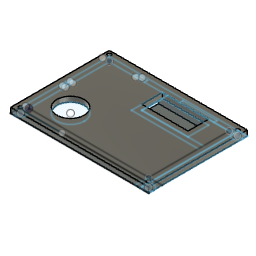
macronoxylid V2 v1 (Autodesk Fusion 360 design; units mm, degrees)
Autodesk Fusion 360 part; units mm, degrees
sketch "Sketch1" plane through (0, 0, 0) normal (0, 0, 1) x (1, 0, 0)
  line L0 (1, 0) -> (69, 0)
  line L1 (0, 1) -> (0, 46)
  line L2 (1, 47) -> (17.5, 47)
  line L3 (17.5, 47) -> (15.35, 47)
  line L4 (70, 1) -> (70, 46)
  line L5 (0, 23.5) -> (0, 25.65)
  line L6 (0, 23.5) -> (0, 21.35)
  line L7 (-1.7, 23.5) -> (-1.7, 25.8)
  line L8 (-1.7, 23.5) -> (-1.7, 21.2)
  line L9 (0, 0) -> (-2.8284, -2.8284)
  line L10 (0, 0) -> (-2, 0) construction
  line L11 (70, 47) -> (72.8284, 49.8284)
  line L12 (70, 47) -> (74, 47) construction
  line L13 (70, 0) -> (72.8284, -2.8284)
  line L14 (0, 47) -> (-2.8284, 49.8284)
  line L15 (0, 47) -> (-4, 47) construction
  line L16 (-2.8284, 49.8284) -> (72.8284, 49.8284)
  line L17 (72.8284, 49.8284) -> (72.8284, -2.8284)
  line L18 (72.8284, -2.8284) -> (-2.8284, -2.8284)
  line L19 (-2.8284, 49.8284) -> (-2.8284, -2.8284)
  line L20 (17.5, 47) -> (69, 47)
  line L21 (41.1957, 48.7475) -> (61.1957, 48.7475)
  line L22 (41.1957, 48.7475) -> (41.1957, 47)
  line L23 (61.1957, 48.7475) -> (61.1957, 47)
  line L24 (17.5, 48.7) -> (14.5, 48.7)
  line L25 (14.5, 48.7) -> (20.5, 48.7)
  line L26 (20.5, 48.7) -> (20.5, 47)
  line L27 (14.5, 48.7) -> (14.5, 47)
  line L28 (-1.7, 23.5) -> (-1.7, 26.5)
  line L29 (-1.7, 26.5) -> (-1.7, 23.5)
  line L30 (-1.7, 23.5) -> (-1.7, 20.5)
  line L31 (-1.7, 20.5) -> (-1.7, 26.5)
  line L32 (0, 26.5) -> (-1.7, 26.5)
  line L33 (-1.7, 20.5) -> (0, 20.5)
  arc A0 (70, 46) -> (69, 47) centre (70, 47) ccw
  arc A1 (1, 47) -> (0, 46) centre (0, 47) ccw
  arc A2 (0, 1) -> (1, 0) centre (0, 0) ccw
  arc A3 (69, 0) -> (70, 1) centre (70, 0) ccw
  line L34 (-2.8284, -2.8284) -> (22.1716, -2.8284)
  circle A4 centre (14.6716, 9.6716) radius 8
  line L35 (70, 47) -> (34, 47)
  line L36 (34, 47) -> (34, 32)
  line L37 (34, 32) -> (70, 32)
  line L38 (34, 32) -> (61, 32)
  line L39 (61, 32) -> (61, 44)
  line L40 (61, 44) -> (34, 44)
  line L41 (34, 44) -> (34, 32)
  line L42 (34, 47) -> (31, 47)
  line L43 (31, 47) -> (31, 29)
  line L44 (31, 29) -> (70, 29)
  line L45 (-2.8284, -2.8284) -> (72.8284, -2.8284)
  line L46 (72.8284, -2.8284) -> (72.8284, -7.8284)
  line L47 (72.8284, -7.8284) -> (-2.8284, -7.8284)
  line L48 (-2.8284, -7.8284) -> (-2.8284, -2.8284)
  line L49 (72.8284, -7.8284) -> (77.8284, -7.8284)
  line L50 (77.8284, -7.8284) -> (77.8284, 49.8284)
  line L51 (77.8284, 49.8284) -> (72.8284, 49.8284)
  line L52 (72.8284, 49.8284) -> (72.8284, -7.8284)
  line L53 (-2.8284, 49.8284) -> (-1.4496, 48.4496)
  circle A5 centre (-0.7071, 47.7071) radius 1.05
  line L54 (69, 47) -> (77.8284, 47)
  line L55 (69, 0) -> (77.8284, 0)
  line L56 (70, 0) -> (70, -7.8284)
  line L57 (0, 1) -> (0, -7.8284)
  line L58 (77.8284, -7.8284) -> (74.9994, -7.8284)
  line L59 (74.9994, -7.8284) -> (74.9994, 49.8284)
  line L60 (77.8284, -7.8284) -> (77.8284, -4.9994)
  line L61 (77.8284, -4.9994) -> (-2.8284, -4.9994)
  circle A6 centre (74.9994, 47) radius 2.829
  circle A7 centre (74.9994, -4.9994) radius 2.829
  circle A8 centre (0, -4.9994) radius 2.829
  circle A9 centre (0, -4.9994) radius 1.05
  circle A10 centre (74.9994, -4.9994) radius 1.05
  circle A11 centre (74.9994, 47) radius 1.05
  dimension "d1" = 70
  dimension "d2" = 47
  dimension "d3" = 17.5
  dimension "d5" = 2.15
  dimension "d23" = 2.15
  dimension "d25" = 1.7
  dimension "d26" = 2.3
  dimension "d27" = 2.3
  dimension "d28" = 45
  dimension "d29" = 4
  dimension "d30" = 4
  dimension "d31" = 45
  dimension "d32" = 4
  dimension "d33" = 45
  dimension "d34" = 4
  dimension "d59" = 6
  dimension "d60" = 3
  dimension "d61" = 3
  dimension "d62" = 2
  dimension "d63" = 2
  dimension "d64" = 2
  dimension "d65" = 2
  dimension "d70" = 20
  dimension "d71" = 11.6328
  dimension "d72" = 25
  dimension "d74" = 16
  dimension "d77" = 36
  dimension "d78" = 15
  dimension "d79" = 27
  dimension "d80" = 12
  dimension "d81" = 3
  dimension "d105" = 5
  dimension "d106" = 5
  dimension "d110" = 2.829
  dimension "d111" = 2.829
  dimension "d112" = 2.1
  dimension "d113" = 2.1
  dimension "d114" = 2.1
  constraint horizontal L0
  constraint coincident L9.start L10.start
  constraint perpendicular L0 L1
  constraint perpendicular L1 L2
  constraint parallel L2 L3
  constraint perpendicular L0 L4
  constraint parallel L1 L5
  constraint parallel L1 L6
  constraint horizontal L10
  constraint horizontal L12
  constraint horizontal L15
  constraint perpendicular L12 L17
  constraint perpendicular L4 L20
  constraint coincident L20 L22.end
  constraint perpendicular L20 L22
  constraint coincident L20 L23.end
  constraint perpendicular L20 L23
  constraint coincident L20 L26.end
  constraint perpendicular L20 L26
  constraint coincident L2 L27.end
  constraint perpendicular L2 L27
  constraint coincident L1 L32.start
  constraint coincident L1 L33.end
  constraint perpendicular L1 L33
  constraint coincident L11.start L12.start
  constraint coincident L14.start L15.start
  constraint coincident L1 L5.start
  constraint coincident L13.start A3.centre
  constraint perpendicular L19 L34
  constraint parallel L20 L35
  constraint perpendicular L35 L36
  constraint coincident L4 L37.end
  constraint perpendicular L4 L37
  constraint horizontal L38
  constraint vertical L39
  constraint horizontal L40
  constraint vertical L41
  constraint perpendicular L36 L42
  constraint perpendicular L38 L43
  constraint coincident L4 L44.end
  constraint perpendicular L4 L44
  constraint horizontal L45
  constraint vertical L46
  constraint horizontal L47
  constraint vertical L48
  constraint horizontal L49
  constraint vertical L50
  constraint horizontal L51
  constraint vertical L52
  constraint parallel L14 L53
  constraint midpoint A1 A5.centre
  constraint coincident L53.end A5
  constraint coincident L50 L54.end
  constraint perpendicular L50 L54
  constraint coincident L50 L55.end
  constraint perpendicular L50 L55
  constraint coincident L47 L56.end
  constraint perpendicular L47 L56
  constraint coincident L47 L57.end
  constraint perpendicular L47 L57
  constraint perpendicular L50 L58
  constraint coincident L51 L59.end
  constraint perpendicular L51 L59
  constraint perpendicular L58 L60
  constraint horizontal L61
  constraint coincident L48 L61.end
  constraint coincident L59 A6.centre
  constraint coincident L54 A6.centre
  constraint coincident L54.end A6
  constraint coincident L59 A7.centre
  constraint coincident L61 A7.centre
  constraint coincident L60.end A7
  constraint coincident L57 A8.centre
  constraint coincident L61 A8.centre
  constraint coincident L57.end A8
  constraint concentric A8 A9
  constraint concentric A7 A10
  constraint concentric A6 A11
  measures "d1" distance of L9.start L13.start
  measures "d2" distance of L9.start L14.start
  measures "d3" distance of L14.start L2.end
  measures "d5" distance of L2.end L3.end
  measures "d23" distance of L5.start L5.end
  measures "d25" distance of L5.start L7.start
  measures "d26" distance of L7.start L7.end
  measures "d27" distance of L7.start L8.end
  measures "d28" angle of L9 L10
  measures "d29" distance of L9.start L9.end
  measures "d30" distance of L11.start L11.end
  measures "d31" angle of L11 L12
  measures "d32" distance of L13.start L13.end
  measures "d33" angle of L14 L15
  measures "d34" distance of L14.start L14.end
  measures "d59" distance of L24.end L25.end
  measures "d60" distance of L7.start L28.end
  measures "d61" distance of L7.start L30.end
  measures "d62" diameter of A0
  measures "d63" diameter of A1
  measures "d64" diameter of A2
  measures "d65" diameter of A3
  measures "d70" horizontal distance of L21.start L21.end
  measures "d71" distance of L17 L23
  measures "d72" distance of L9.end L34.end
  measures "d74" diameter of A4
  measures "d77" distance of L11.start L35.end
  measures "d78" distance of L35.end L36.end
  measures "d79" distance of L36.end L38.end
  measures "d80" distance of L36.end L40.end
  measures "d81" distance of L35.end L42.end
  measures "d105" distance of L9.end L47.end
  measures "d106" distance of L46.end L49.end
  measures "d110" distance of L49.end L58.end
  measures "d111" distance of L49.end L60.end
  measures "d112" diameter of A9
  measures "d113" diameter of A10
  measures "d114" diameter of A11
sketch "Sketch2" plane through (0, 49.8284, 0) normal (0, 1, 0) x (-1, 0, 0)
  line L0 (-72.8284, 0) -> (2.8284, 0)
  line L1 (2.8284, 0) -> (2.8284, 28)
  line L2 (2.8284, 28) -> (-72.8284, 28)
  line L3 (-72.8284, 28) -> (-72.8284, 0)
  line L4 (-72.8284, 0) -> (-41.8284, 0)
  line L5 (-41.8284, 0) -> (-51.0284, 0)
  line L6 (-51.0284, 0) -> (-51.0284, 17)
  line L7 (-51.0284, 17) -> (-55.0284, 17)
  line L8 (-55.0284, 17) -> (-47.0284, 17)
  line L9 (-47.0284, 17) -> (-47.0284, 14)
  line L10 (-47.0284, 14) -> (-55.0284, 14)
  line L11 (-55.0284, 14) -> (-55.0284, 17)
  dimension "d49" = 31
  dimension "d50" = 9.2
  dimension "d51" = 17
  dimension "d52" = 4
  dimension "d53" = 8
  dimension "d54" = 3
  constraint coincident L0.start L3.end
  constraint perpendicular L3 L4
  constraint parallel L4 L5
  constraint perpendicular L4 L6
  constraint perpendicular L6 L7
  constraint horizontal L8
  constraint vertical L9
  constraint horizontal L10
  constraint vertical L11
  measures "d49" distance of L0.start L4.end
  measures "d50" distance of L4.end L5.end
  measures "d51" distance of L5.end L6.end
  measures "d52" distance of L6.end L7.end
  measures "d53" distance of L7.end L8.end
  measures "d54" distance of L7.end L10.end
extrude "Extrude9" add sketch "Sketch1" along normal blind 3 contours L0 L1 L2 L3 L4 L5 L6 L20 A1 A2 A3 L43 L44 A5 L55 L57 | L0 L18 A2 A3 L34 L45 L56 L57 A8 | A3 L55 L56 | L9 L18 A2 L34 L45 L57 A8 | L9 A2 L57 | L13 A3 L56 | L13 L18 A3 L45 L56 | L13 A3 L55 | L9 A2 L57 | L1 L7 L8 L9 L14 L19 L28 L29 L30 L31 L32 L33 A1 A2 L53 A5 | L18 L34 L45 L57 A8 | L18 L34 L45 L57 A8 | L13 L17 A3 L52 L55 | L4 L17 A0 A3 L52 L54 L55 A6 | L2 L11 L14 L16 L20 L21 L22 L23 L24 L25 L26 L27 A0 A1 L35 L42 L53 A5 | L17 L52 L54 A6 | L14 A1 A5 | L14 A1 A5 | L11 L17 A0 L52 L54 A6 | L17 L52 L54 A6 | A1 A5
extrude "Extrude11" add sketch "Sketch1" along normal blind 3 and the other way blind 7 contours L4 L20 L36 L37 L38 L41 L42 L43 L44 | L4 L20 A0 L35 L36 L37 L39 L40 L54 | L11 A0 L54 | L36 L37 L38 L39 L40 L41
sketch "Sketch3" plane through (31, 0, 0) normal (-1, 0, 0) x (0, -1, 0)
  line L0 (-29, 0) -> (-47, 0)
  line L1 (-47, 0) -> (-47, -7)
  line L2 (-47, -7) -> (-29, -7)
  line L3 (-29, -7) -> (-29, 0)
  line L4 (-29, 0) -> (-31.25, 0)
  line L5 (-31.25, 0) -> (-31.25, -4.5)
  line L6 (-31.25, -4.5) -> (-44.75, -4.5)
  line L7 (-44.75, -4.5) -> (-44.75, 0)
  line L8 (-44.75, 0) -> (-31.25, 0)
  dimension "d92" = 2.25
  dimension "d93" = 4.5
  dimension "d94" = 13.5
  constraint coincident L0.start L3.end
  constraint perpendicular L3 L4
  constraint perpendicular L4 L5
  constraint perpendicular L5 L6
  constraint coincident L0 L7.end
  constraint perpendicular L0 L7
  measures "d92" distance of L0.start L4.end
  measures "d93" distance of L4.end L5.end
  measures "d94" distance of L5.end L6.end
extrude "Extrude12" cut sketch "Sketch3" against normal blind 30 contours L0 L5 L6 L7 L8
extrude "Extrude13" cut sketch "Sketch1" along normal blind 3 contours L36 L37 L38 L39 L40 L41
extrude "Extrude14" add sketch "Sketch1" along normal blind 3 contours L11 A0 L35 L54
extrude "Extrude15" cut sketch "Sketch3" against normal blind 36 contours L0 L5 L6 L7 L8
extrude "Extrude16" add sketch "Sketch1" along normal blind 3 contours L1 L5 L6 L7 L8 L28 L29 L30 L31 L32 L33 | L2 L3 L20 L24 L25 L26 L27 | L20 L21 L22 L23 L35
extrude "Extrude17" add sketch "Sketch1" along normal blind 3 contours L18 L34 L45 L56 L61 A8 | L18 L45 L46 L52 L56 L61 A7 | L18 L34 L45 L48 A8 | L18 L34 L45 L57 L61 A8 A9 | L18 L34 L45 L57 L61 A8 A9 | L17 L46 L52 L55 L59 A7 | L46 L47 L52 L56 L61 A7 | L47 L56 L61 A8 | L17 L52 L55 L59 A6 | L47 L48 A8 | L57 L61 A8 A9 | L57 L61 A9 | L57 L61 A9 | L57 L61 A8 A9 | L46 L52 L59 L61 A7 A10 | L46 L52 L61 A7 | L46 L52 L61 A7 | L17 L52 L54 L59 A6 A11 | L50 L55 L59 A6 | L50 L55 L59 A7 | L17 L51 L52 A6 | L57 L61 A9 | L57 L61 A9 | L46 L52 L59 L61 A7 A10 | L59 L61 A7 A10 | L46 L49 L52 A7 | L17 L52 L54 L59 A6 A11 | L54 L59 A6 A11 | L54 L59 A6 A11 | L50 L51 A6 | L59 L61 A10 | L59 L61 A10 | L59 L61 A10 | L59 L61 A7 A10 | L49 L50 L58 L60 A7 | L54 L59 A11 | L54 L59 A11 | L54 L59 A11 | L54 L59 A11 | L59 L61 A10
extrude "Extrude18" cut sketch "Sketch1" along normal blind 3 contours L57 L61 A9 | L57 L61 A9 | L14 A1 A5 | L14 A1 A5 | L57 L61 A9 | L57 L61 A9 | A1 A5 | L59 L61 A10 | L59 L61 A10 | L59 L61 A10 | L54 L59 A11 | L54 L59 A11 | L54 L59 A11 | L54 L59 A11 | L59 L61 A10
equation "d3 = ( 35 / 2 ) * 1 mm"
equation "d50 = ( 18.4 / 2 ) * 1 mm"
equation "d71 = 12.6327619515 mm - 1 mm"
equation "d77 = 33 mm + 3 mm"
equation "d78 = 12 mm + 3 mm"
equation "d79 = 36.000 mm - 9 mm"
equation "d80 = 15.000 mm - 3 mm"
equation "d101 = 0.00 mm - 36 mm"
